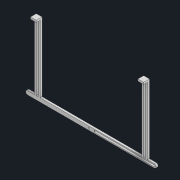
# Autodesk Inventor part: Bancada
Saved by Autodesk Inventor 2021 (Build 250183000, 183)
## iProperties
Created: 2021-04-19
Part Number: Bancada
Material: Genérico
Document SubType Name: Modeling
Designer: carlo
Density: 1 g/cm^3
Appearance: Valor por defecto
Author: carlo
Autodesk Inventor part; units mm, degrees
ref_plane "YZ Plane" through (0, 0, 0) normal (1, 0, 0) x (0, 1, 0)
ref_plane "XZ Plane" through (0, 0, 0) normal (0, 1, 0) x (-1, 0, 0)
ref_plane "XY Plane" through (0, 0, 0) normal (0, 0, 1) x (1, 0, 0)
sketch "Boceto1" plane through (0, 0, 0) normal (0, 0, 1) x (1, 0, 0)
  arc A0 (165, -5) -> (165, 5) centre (165, 0) ccw
  arc A1 (165, -2.5) -> (165, 2.5) centre (165, 0) ccw
  line L0 (5, -5) -> (165, -5)
  line L1 (165, -2.5) -> (8, -2.5)
  line L2 (8, -2.5) -> (8, 2.5)
  line L3 (8, 2.5) -> (165, 2.5)
  line L4 (165, 2.5) -> (165, -2.5)
  line L5 (140, 5) -> (142.5, 5)
  line L6 (142.5, 5) -> (137.5, 5)
  line L7 (137.5, 5) -> (137.5, 180)
  line L8 (142.5, 180) -> (142.5, 5)
  line L9 (132.5, 185) -> (147.5, 185)
  line L10 (147.5, 185) -> (147.5, 5)
  line L11 (142.5, 5) -> (137.5, 5)
  line L12 (132.5, 5) -> (132.5, 185)
  line L13 (137.5, 180) -> (142.5, 180)
  line L14 (147.5, 5) -> (165, 5)
  line L15 (0, 5) -> (132.5, 5)
  line L16 (137.5, 5) -> (142.5, 5)
  line L17 (0, -2.5) -> (0, 2.5)
  arc A2 (-165, 5) -> (-165, -5) centre (-165, 0) ccw
  line L18 (5, -5) -> (-165, -5)
  line L19 (-140, 5) -> (-142.5, 5)
  line L20 (-142.5, 5) -> (-137.5, 5)
  line L21 (-137.5, 5) -> (-137.5, 180)
  line L22 (-142.5, 180) -> (-142.5, 5)
  line L23 (-132.5, 185) -> (-147.5, 185)
  line L24 (-147.5, 185) -> (-147.5, 5)
  line L25 (-142.5, 5) -> (-137.5, 5)
  line L26 (-132.5, 5) -> (-132.5, 185)
  line L27 (-137.5, 180) -> (-142.5, 180)
  line L28 (-147.5, 5) -> (-165, 5)
  line L29 (0, 5) -> (-132.5, 5)
  line L30 (-137.5, 5) -> (-142.5, 5)
  line L31 (147.5, 9.2098) -> (160, 9.2098) construction
  line L32 (160, 9.2098) -> (165, 9.2098) construction
  line L33 (132.5, 17.1248) -> (8, 17.1248) construction
  line L34 (0, 0) -> (-5, 0) construction
  circle A3 centre (-5, 0) radius 2.5
  dimension "d2" = 10
  dimension "d3" = 5
  dimension "d13" = 15
  dimension "d17" = 180
  dimension "d18" = 175
  dimension "d29" = 160
  dimension "d31" = 10
  dimension "d33" = 5
  dimension "d34" = 5
  constraints: 70 end point, 12 symmetric about line, 8 parallel, 6 horizontal, 6 point on circle, 4 centre point, 4 perpendicular, 3 point on line, 3 tangent, 2 coincident, 2 vertical, 1 other
  measures "d2" diameter of A0
  measures "d3" diameter of A1
  measures "d13" distance of L10.end L12.start
  measures "d17" distance of L12.start L9.start
  measures "d18" distance between parallel lines of L15 L13
  measures "d29" distance of L0.start L0.end
  measures "d31" distance between parallel lines of L29 L18
  measures "d33" distance of L34.start L34.end
  measures "d34" diameter of A3
extrude "Extrusión1" add sketch "Boceto1" along normal blind 5
sketch "Sketch4" plane through (0, 0, 5) normal (0, 0, 1) x (1, 0, 0)
  line L0 (-132.5, 185) -> (-147.5, 185) projected
  line L1 (-132.5, 5) -> (-132.5, 185) projected
  line L2 (-147.5, 185) -> (-132.5, 185)
  line L3 (-132.5, 185) -> (-132.5, 180)
  line L4 (-132.5, 180) -> (-147.5, 180)
  line L5 (-147.5, 180) -> (-147.5, 185)
  arc A0 (165, -5) -> (165, 5) centre (165, 0) ccw projected
  line L6 (165, 5) -> (147.5, 5) projected
  line L7 (147.5, 5) -> (147.5, 185) projected
  line L8 (147.5, 185) -> (132.5, 185) projected
  line L9 (132.5, 185) -> (132.5, 5) projected
  line L10 (132.5, 5) -> (-132.5, 5) projected
  line L11 (-132.5, 5) -> (-132.5, 185) projected
  line L12 (-132.5, 185) -> (-147.5, 185) projected
  line L13 (-147.5, 185) -> (-147.5, 5) projected
  line L14 (-147.5, 5) -> (-165, 5) projected
  arc A1 (-165, 5) -> (-165, -5) centre (-165, 0) ccw projected
  line L15 (-165, -5) -> (165, -5) projected
  line L16 (-142.5, 5) -> (-142.5, 180) projected
  line L17 (-142.5, 180) -> (-137.5, 180) projected
  line L18 (-137.5, 180) -> (-137.5, 5) projected
  line L19 (-137.5, 5) -> (-142.5, 5) projected
  line L20 (165, -2.5) -> (8, -2.5) projected
  line L21 (8, -2.5) -> (8, 2.5) projected
  line L22 (8, 2.5) -> (165, 2.5) projected
  arc A2 (165, -2.5) -> (165, 2.5) centre (165, 0) ccw projected
  line L23 (142.5, 180) -> (142.5, 5) projected
  line L24 (142.5, 5) -> (137.5, 5) projected
  line L25 (137.5, 5) -> (137.5, 180) projected
  line L26 (137.5, 180) -> (142.5, 180) projected
  line L27 (132.5, 185) -> (147.5, 185)
  line L28 (147.5, 185) -> (147.5, 180)
  line L29 (147.5, 180) -> (132.5, 180)
  line L30 (132.5, 180) -> (132.5, 185)
  point P0 (0, 0)
  point P1 (142.5, 180)
  dimension "d26" = 5
  constraints: 16 end point, 4 parallel, 2 horizontal, 2 perpendicular, 2 point on line
  measures "d26" distance of L2.end L3.end
extrude "Extrusion3" add sketch "Sketch4" along normal blind 10 contours L1 L4 L5 L0 | L9 L8 L7 L29 L26
